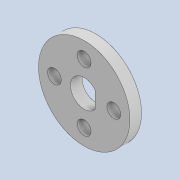
# Autodesk Inventor part: ForearmDHub
Saved by Autodesk Inventor 2020.4 (Build 244396010, 396A)
## iProperties
Created: 2021-09-16
Part Number: ForearmDHub
Material: Generic
Document SubType Name: Sheet Metal
Designer: Val
Density: 1 g/cm^3
Sheet Metal Rule: Default
Appearance: Default
Author: Val
Autodesk Inventor part; units mm, degrees
ref_plane "YZ Plane" through (0, 0, 0) normal (1, 0, 0) x (0, 1, 0)
ref_plane "XZ Plane" through (0, 0, 0) normal (0, 1, 0) x (-1, 0, 0)
ref_plane "XY Plane" through (0, 0, 0) normal (0, 0, 1) x (1, 0, 0)
sketch "Sketch1" plane through (0, 0, 0) normal (0, 0, 1) x (1, 0, 0)
  circle A0 centre (0, 0) radius 10
  arc A1 (2.4, 1.8) -> (2.4, -1.8) centre (0, 0) ccw
  line L0 (-10, 0) -> (10, 0) construction
  line L1 (0, 10) -> (0, -10) construction
  circle A2 centre (0, 0) radius 6.5 construction
  circle A3 centre (-6.5, 0) radius 1.5
  circle A4 centre (0, 6.5) radius 1.5
  circle A5 centre (0, -6.5) radius 1.5
  circle A6 centre (6.5, 0) radius 1.5
  line L2 (-3, 0) -> (0, 0) construction
  line L3 (2.4, 1.8) -> (2.4, -1.8)
  arc A7 (3, 0) -> (2.4, 1.8) centre (0, 0) ccw construction
  arc A8 (2.4, -1.8) -> (3, 0) centre (0, 0) ccw construction
  dimension "d0" = 6
  dimension "d1" = 20
  dimension "d2" = 3
  dimension "d3" = 3.5
  dimension "d4" = 3
  dimension "d5" = 3
  dimension "d6" = 3
  dimension "d7" = 5.4
  measures "d0" diameter of A1
  measures "d1" diameter of A0
  measures "d2" diameter of A3
  measures "d3" radial gap between concentric circles of A0 A2
  measures "d4" diameter of A4
  measures "d5" diameter of A5
  measures "d6" diameter of A6
  measures "d7" distance from line of L2.start L3
extrude "Plate1" add sketch "Sketch1" along normal blind 2.54
equation "\"d8\" = Thickness"
equation "\"BendRadius\" = Thickness"
equation "\"BendReliefWidth\" = Thickness"
equation "\"BendReliefDepth\" = 0.5 * Thickness"
equation "\"CornerReliefSize\" = 4 * Thickness"
equation "\"MinimumRemnant\" = 2 * Thickness"
equation "\"TransitionRadius\" = BendRadius"
equation "\"JacobiRadiusSize\" = BendRadius"
equation "\"GapSize\" = Thickness"
equation "\"Thickness\" = 2.54"
body "Solid1"
